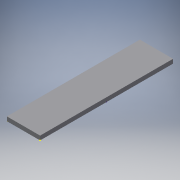
# Autodesk Inventor part: Drive Motor Plate
Saved by Autodesk Inventor 2017 (Build 210142000, 142)
## iProperties
Created: 2016-12-03
Part Number: Drive Motor Plate
Material: Generic
Document SubType Name: Modeling
Designer: Aditya
Density: 1 g/cm^3
Appearance: Default
Author: Aditya
Autodesk Inventor part; units mm, degrees
ref_plane "YZ Plane" through (0, 0, 0) normal (1, 0, 0) x (0, 1, 0)
ref_plane "XZ Plane" through (0, 0, 0) normal (0, 1, 0) x (-1, 0, 0)
ref_plane "XY Plane" through (0, 0, 0) normal (0, 0, 1) x (1, 0, 0)
sketch "Sketch1" plane through (0, 0, 0) normal (0, 1, 0) x (-1, 0, 0)
  line L0 (0, 0) -> (0, -101.6)
  line L1 (0, -101.6) -> (25.4, -101.6)
  line L2 (25.4, -101.6) -> (25.4, 0)
  line L3 (25.4, 0) -> (0, 0)
  dimension "d0" = 101.6
  dimension "d1" = 25.4
  constraints: 8 end point, 2 perpendicular, 2 vertical
  measures "d0" distance of L0.start L0.end
  measures "d1" distance of L0.end L1.end
extrude "Extrusion1" add sketch "Sketch1" along normal blind 3.175
sketch "Sketch2" plane through (0, 0, 0) normal (0, -1, 0) x (1, 0, 0)
  line L0 (-25.4, -101.6) -> (-25.4, 0) projected
  line L1 (-25.4, -50.8) -> (0, -50.8)
  point P0 (0, 0)
  constraints: 2 end point, 1 horizontal, 1 midpoint
sketch "Sketch3" plane through (0, 3.175, 0) normal (0, 1, 0) x (1, 0, 0)
  line L0 (0, 0) -> (0, 101.6) projected
  line L1 (0, 50.8) -> (-25.4, 50.8)
  line L2 (-25.4, 101.6) -> (-25.4, 0) projected
  line L3 (-25.4, 0) -> (0, 0) projected
  line L4 (-12.7, 0) -> (-12.7, 101.5312)
  constraints: 4 end point, 3 midpoint, 1 vertical
sketch "Sketch4" plane through (0, 3.175, 0) normal (0, 1, 0) x (1, 0, 0)
  circle A0 centre (-12.7, 18.8) radius 1.85 projected
  circle A1 centre (-12.7, 82.8) radius 1.85 projected
  point P0 (0, 0)
extrude "Extrusion2" cut sketch "Sketch4" against normal blind 23.8125
body "Solid1"
